LiPo 11Wh (Autodesk Fusion 360 design; units mm, degrees)
Autodesk Fusion 360 part; units mm, degrees
sketch "Sketch1" plane through (0, 0, 0) normal (0, 0, 1) x (1, 0, 0)
  line L0 (8.75, 37.75) -> (-8.75, 37.75)
  line L1 (-8.75, 37.75) -> (-8.75, -37.75)
  line L2 (-8.75, -37.75) -> (8.75, -37.75)
  line L3 (8.75, -37.75) -> (8.75, 37.75)
  line L4 (8.75, 37.75) -> (-8.75, -37.75) construction
  line L5 (-8.75, 37.75) -> (8.75, -37.75) construction
  dimension "d1" = 17.5
  dimension "d2" = 75.5
  constraint horizontal L0
  constraint perpendicular L0 L1
  constraint parallel L0 L2
  constraint parallel L1 L3
  constraint coincident L4 origin
  constraint coincident L5 origin
  measures "d1" distance of L1.end L2.end
  measures "d2" distance of L0.end L1.end
extrude "Extrude1" add sketch "Sketch1" along normal blind 30
fillet "Fillet1" radius 2.5 4 edges at (8.75, 0, 30) (-8.75, 0, 30) (8.75, 0, 0) (-8.75, 0, 0)
sketch "Sketch2" plane through (0, -37.75, 0) normal (0, -1, 0) x (1, 0, 0)
  arc A0 (-8.75, 2.5) -> (-6.25, 0) centre (-6.25, 2.5) ccw
  line L0 (-6.25, 0) -> (6.25, 0)
  arc A1 (6.25, 0) -> (8.75, 2.5) centre (6.25, 2.5) ccw
  line L1 (8.75, 2.5) -> (8.75, 27.5)
  arc A2 (8.75, 27.5) -> (6.25, 30) centre (6.25, 27.5) ccw
  line L2 (6.25, 30) -> (-6.25, 30)
  arc A3 (-6.25, 30) -> (-8.75, 27.5) centre (-6.25, 27.5) ccw
  line L3 (-8.75, 27.5) -> (-8.75, 2.5)
  line L4 (-5.5, 3) -> (5.5, 3)
  line L5 (5.5, 3) -> (5.5, 0)
  line L6 (5.5, 0) -> (-5.5, 0)
  line L7 (-5.5, 0) -> (-5.5, 3)
  dimension "d7" = 11
  dimension "d8" = 3
  constraint horizontal L4
  constraint vertical L5
  constraint horizontal L6
  constraint vertical L7
  constraint midpoint L0 L6
  measures "d7" distance of L4.start L4.end
  measures "d8" distance of L4 L6
extrude "Extrude2" add sketch "Sketch2" along normal blind 12 contours L0 L4 L5 L6 L7
